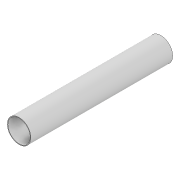
# Autodesk Inventor part: Φ35mm_Pipe
Saved by Autodesk Inventor 2020.1 (Build 241239000, 239)
## iProperties
Created: 2020-10-05
Part Number: Φ35mm_Pipe
Material: 一般
Document SubType Name: Modeling
Designer: kenta iguchi
Density: 1 g/cm^3
Appearance: 既定
Author: kenta iguchi
Autodesk Inventor part; units mm, degrees
ref_plane "YZ Plane" through (0, 0, 0) normal (1, 0, 0) x (0, 1, 0)
ref_plane "XZ Plane" through (0, 0, 0) normal (0, 1, 0) x (-1, 0, 0)
ref_plane "XY Plane" through (0, 0, 0) normal (0, 0, 1) x (1, 0, 0)
sketch "スケッチ1" plane through (0, 0, 0) normal (0, 0, 1) x (1, 0, 0)
  circle A0 centre (0, 0) radius 17.5
  circle A1 centre (0, 0) radius 16.5
  dimension "d0" = 35
  dimension "d1" = 1
  constraints: 2 centre point, 1 coincident
  measures "d0" diameter of A0
  measures "d1" radial gap between concentric circles of A0 A1
extrude "押し出し1" add sketch "スケッチ1" along normal blind 210
